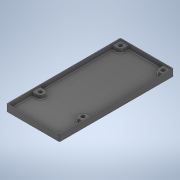
# Autodesk Inventor part: J120_cover
Saved by Autodesk Inventor 2020 (Build 240168000, 168)
## iProperties
Created: 2021-08-15
Part Number: J120_cover
Material: アセタール樹脂、黒
Document SubType Name: Modeling
Designer: Masato Kubotera
Density: 1.425 g/cm^3
Appearance: 滑らか - 黒
Description: PLA
Author: Masato Kubotera
Title: Circuit_protection_02
Autodesk Inventor part; units mm, degrees
ref_plane "YZ Plane" through (0, 0, 0) normal (1, 0, 0) x (0, 1, 0)
ref_plane "XZ Plane" through (0, 0, 0) normal (0, 1, 0) x (-1, 0, 0)
ref_plane "XY Plane" through (0, 0, 0) normal (0, 0, 1) x (1, 0, 0)
sketch "スケッチ1" plane through (0, 0, 0) normal (0, 0, 1) x (1, 0, 0)
  line L0 (-26.2, 56.2) -> (26.2, 56.2)
  line L1 (26.2, 56.2) -> (26.2, -56.2)
  line L2 (26.2, -56.2) -> (-26.2, -56.2)
  line L3 (-26.2, -56.2) -> (-26.2, 56.2)
  line L4 (-26.2, 56.2) -> (26.2, -56.2) construction
  line L5 (26.2, 56.2) -> (-26.2, -56.2) construction
  line L6 (-25.2, 55.2) -> (25.2, 55.2)
  line L7 (25.2, 55.2) -> (25.2, -55.2)
  line L8 (25.2, -55.2) -> (-25.2, -55.2)
  line L9 (-25.2, -55.2) -> (-25.2, 55.2)
  line L10 (-25.2, 55.2) -> (25.2, -55.2) construction
  line L11 (25.2, 55.2) -> (-25.2, -55.2) construction
  line L12 (-25, 55) -> (25, 55) construction
  line L13 (25, 55) -> (25, -55) construction
  line L14 (25, -55) -> (-25, -55) construction
  line L15 (-25, -55) -> (-25, 55) construction
  line L16 (-25, 55) -> (25, -55) construction
  line L17 (25, 55) -> (-25, -55) construction
  line L18 (-26.25, 56.25) -> (26.25, 56.25) construction
  line L19 (26.25, 56.25) -> (26.25, -56.25) construction
  line L20 (26.25, -56.25) -> (-26.25, -56.25) construction
  line L21 (-26.25, -56.25) -> (-26.25, 56.25) construction
  line L22 (-26.25, 56.25) -> (26.25, -56.25) construction
  line L23 (26.25, 56.25) -> (-26.25, -56.25) construction
  circle A0 centre (-21, 51) radius 1.75
  circle A1 centre (-21, -28) radius 1.75
  line L24 (0, 56.25) -> (0, -56.25) construction
  circle A2 centre (21, 51) radius 1.75
  circle A3 centre (21, -28) radius 1.75
  arc A4 (-21, -32) -> (-21, -24) centre (-21, -28) ccw
  line L25 (-21, 47) -> (-25.2, 47)
  line L26 (-17, 51) -> (-17, 55.2)
  arc A5 (-21, 47) -> (-17, 51) centre (-21, 51) ccw
  line L27 (-21, -24) -> (-25.2, -24)
  line L28 (-21, -32) -> (-25.2, -32)
  arc A6 (21, -24) -> (21, -32) centre (21, -28) ccw
  line L29 (21, 47) -> (25.2, 47)
  line L30 (17, 51) -> (17, 55.2)
  arc A7 (17, 51) -> (21, 47) centre (21, 51) ccw
  line L31 (21, -24) -> (25.2, -24)
  line L32 (21, -32) -> (25.2, -32)
  point P0 (0, 0)
  dimension "d0" = 50
  dimension "d1" = 110
  dimension "d2" = 0.2
  dimension "d4" = 0.2
  dimension "d8" = 1
  dimension "d10" = 1
  dimension "d11" = 112.5
  dimension "d12" = 0.05
  dimension "d13" = 0.05
  dimension "d14" = 52.5
  dimension "d15" = 3.5
  dimension "d16" = 4
  dimension "d17" = 4
  dimension "d18" = 3.5
  dimension "d19" = 4
  dimension "d20" = 83
  dimension "d22" = 8
  dimension "d31" = 4
  constraints: 66 end point, 12 symmetric about line, 10 midpoint, 8 centre point, 8 parallel, 8 perpendicular, 8 point on circle, 4 horizontal, 4 point on line, 4 tangent, 2 coincident, 4 other
  measures "d0" distance of L12.start L12.end
  measures "d1" distance of L12.end L13.end
  measures "d2" horizontal distance of L12.start L6.start
  measures "d4" horizontal distance of L12.start L6.start
  measures "d8" horizontal distance of L6.start L0.start
  measures "d10" horizontal distance of L6.start L0.start
  measures "d11" distance of L19.end L18.end
  measures "d12" horizontal distance of L0.start L18.start
  measures "d13" horizontal distance of L0.start L18.start
  measures "d14" distance of L18.start L18.end
  measures "d15" diameter of A0
  measures "d16" horizontal distance of A0.centre L12.start
  measures "d17" horizontal distance of A0.centre L12.start
  measures "d18" diameter of A1
  measures "d19" horizontal distance of L12.start A1.centre
  measures "d20" vertical distance of A1.centre L12.start
  measures "d22" diameter of A4
  measures "d31" radius of A5
extrude "押し出し1" add sketch "スケッチ1" along normal blind 4.8 contours L0 L1 L2 L3
extrude "押し出し2" add sketch "スケッチ1" against normal blind 1.4 contours L0 L1 L2 L3 | L6 L26 A5 L25 L9 | L6 L30 A7 L29 L7 L31 A6 L32 L8 L9 L28 A4 L27 L25 A5 L26 | L6 L7 L29 A7 L30 | L27 A4 L28 L9 | L7 L32 A6 L31
extrude "押し出し3" add sketch "スケッチ1" along normal blind 3.6 contours L6 L26 A5 L25 L9 | L6 L7 L29 A7 L30 | L27 A4 L28 L9 | L7 L32 A6 L31
fillet "フィレット1" radius 1 4 edges at (-26.2, -56.2, 1.7) (26.2, -56.2, 1.7) (26.2, 56.2, 1.7) (-26.2, 56.2, 1.7)
fillet "フィレット2" radius 1 26 edges at (-25.2, 47, 1.8) (-17, 55.2, 1.8) (-25.2, 11.5, 0) (-18.1716, 48.1716, 0) (-17, 53.1, 0) (-23.1, 47, 0) (0, 55.2, 0) (17, 53.1, 0) (23.1, 47, 0) (18.1716, 48.1716, 0) (17, 55.2, 1.8) (25.2, 47, 1.8) (25.2, 11.5, 0) (25.2, -32, 1.8) (23.1, -24, 0) (23.1, -32, 0) (17, -28, 0) (25.2, -43.6, 0) (-23.1, -32, 0) (-23.1, -24, 0) (-17, -28, 0) (0, -55.2, 0) (-25.2, -43.6, 0) (-25.2, -32, 1.8) (-25.2, -24, 1.8) (25.2, -24, 1.8)
equation "\"d4\" = d2"
equation "\"d13\" = d12"
equation "\"d17\" = d16"
equation "\"d18\" = d15"
equation "\"d19\" = d17"
equation "\"d22\" = 2 * d31"
